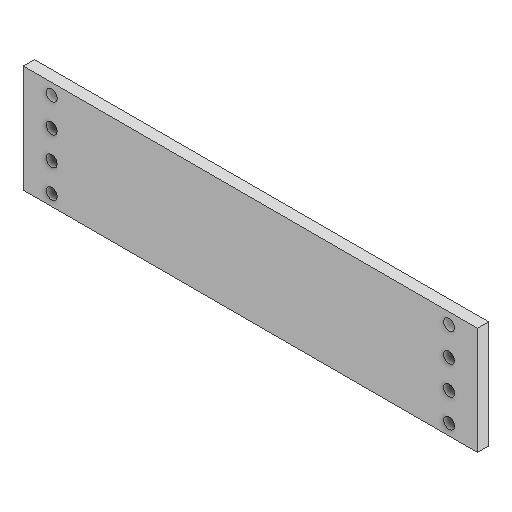
# Autodesk Inventor part: Chapa Guia - Elevador
Saved by Autodesk Inventor 2025.3 (Build 293356000, 356)
## iProperties
Created: 2026-05-13
Part Number: Chapa Guia - Elevador
Material: Genérico
Document SubType Name: Modeling
Designer: djair.oliveira
Density: 1 g/cm^3
Appearance: Padrão
Author: djair.oliveira
Autodesk Inventor part; units mm, degrees
ref_plane "YZ Plane" through (0, 0, 0) normal (1, 0, 0) x (0, 1, 0)
ref_plane "XZ Plane" through (0, 0, 0) normal (0, 1, 0) x (-1, 0, 0)
ref_plane "XY Plane" through (0, 0, 0) normal (0, 0, 1) x (1, 0, 0)
sketch "Esboço1" plane through (0, 0, 0) normal (0, 0, 1) x (1, 0, 0)
  line L0 (101.6, -24.05) -> (-101.6, -24.05)
  line L1 (-101.6, -24.05) -> (-101.6, 24.05)
  line L2 (-101.6, 24.05) -> (101.6, 24.05)
  line L3 (101.6, 24.05) -> (101.6, -24.05)
  line L4 (101.6, -24.05) -> (-101.6, 24.05) construction
  line L5 (-101.6, -24.05) -> (101.6, 24.05) construction
  circle A0 centre (-88.9, 6.35) radius 2.5
  circle A1 centre (-88.9, -6.35) radius 2.5
  circle A2 centre (-88.9, 19.05) radius 2.5
  circle A3 centre (-88.9, -19.05) radius 2.5
  line L6 (0, 0) -> (0, 24.05)
  line L7 (-101.6, -24.05) -> (101.6, 24.05) construction
  line L8 (101.6, -24.05) -> (-101.6, 24.05) construction
  circle A4 centre (88.9, 6.35) radius 2.5
  circle A5 centre (88.9, -6.35) radius 2.5
  circle A6 centre (88.9, 19.05) radius 2.5
  circle A7 centre (88.9, -19.05) radius 2.5
  dimension "d0" = 203.2
  dimension "d1" = 5
  dimension "d2" = 12.7
  dimension "d3" = 12.7
  dimension "d4" = 12.7
  dimension "d5" = 12.7
  dimension "d6" = 5
  dimension "d7" = 5
  constraints: 18 end point, 8 centre point, 8 symmetric about line, 3 equal radius, 3 midpoint, 3 vertical alignment, 2 parallel, 1 horizontal, 1 perpendicular, 4 other
  measures "d0" distance of L1.end L2.end
  measures "d1" diameter of A1
  measures "d2" distance of A0.centre A1.centre
  measures "d3" distance of A3.centre A1.centre
  measures "d4" distance of A2.centre A0.centre
  measures "d5" distance from line of L1 A2.centre
  measures "d6" distance from line of A2.centre L2
  measures "d7" distance from line of A3.centre L0
extrude "Extrusão1" add sketch "Esboço1" along normal blind 5
equation "\"d3\" = d2"
equation "\"d4\" = d2"
equation "\"d7\" = d6"
